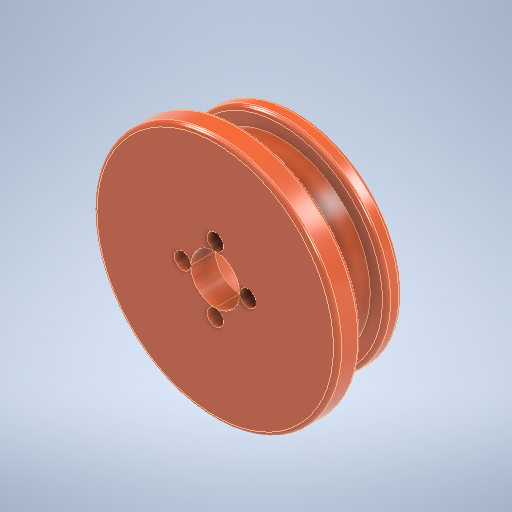
# Autodesk Inventor part: Steering Gear Plate
Saved by Autodesk Inventor 2025.2 (Build 292293000, 293)
## iProperties
Created: 2025-02-06
Part Number: Steering Gear Plate
Material: Generic
Document SubType Name: Modeling
Designer: eason
Density: 1 g/cm^3
Appearance: Smooth - Light Orange
Author: eason
Autodesk Inventor part; units mm, degrees
ref_plane "YZ Plane" through (0, 0, 0) normal (1, 0, 0) x (0, 1, 0)
ref_plane "XZ Plane" through (0, 0, 0) normal (0, 1, 0) x (-1, 0, 0)
sketch "Sketch1" plane through (0, 0, 0) normal (0, 0, 1) x (1, 0, 0)
  circle A0 centre (0, 0) radius 15
  circle A1 centre (0, 0) radius 3
  circle A2 centre (0, 0) radius 5
  circle A3 centre (4, 0) radius 1
  circle A4 centre (-4, 0) radius 1
  line L0 (-21, 0) -> (21, 0) projected
  circle A5 centre (0, 4) radius 1
  circle A6 centre (0, -4) radius 1
  line L1 (0, -21) -> (0, 21) projected
  point P0 (-5, 0)
  point P1 (-3, 0)
  point P2 (3, 0)
  point P3 (5, 0)
  point P4 (0, -5)
  point P5 (0, -3)
  point P6 (0, 3)
  point P7 (0, 5)
  dimension "d0" = 30
  dimension "d1" = 6
  dimension "d2" = 10
  constraints: 8 tangent, 7 centre point, 4 point on line, 3 coincident
  measures "d0" diameter of A0
  measures "d1" diameter of A1
  measures "d2" diameter of A2
extrude "Extrusion1" add sketch "Sketch1" along normal blind 3 contours L0 A2 L1 A0 | A0 L1 A2 L0 | L1 A2 L0 A0 | A0 L0 A2 L1 | A3 A1 A5 A2 | A2 A6 A1 A3 | A5 A1 A4 A2 | A2 A4 A1 A6
ref_plane "Work Plane1" through (0, 0, 1.5) normal (0, 0, 1) x (1, 0, 0)
sketch "Sketch5" plane through (0, 0, 0) normal (0, 0, -1) x (-1, 0, 0)
  line L0 (0, 0) -> (-5.2212, -14.062) construction
  circle A0 centre (0, 0) radius 15 projected
  line L1 (0, -21) -> (0, 21) projected
  circle A1 centre (-4.351, -11.7183) radius 2.5
  arc A2 (-3, 0) -> (3, 0) centre (0, 0) ccw projected
  arc A3 (0.0912, -10.9996) -> (-7.2478, -8.2746) centre (-4.351, -11.7183) ccw
  arc A4 (0.0912, -10.9996) -> (-7.2478, -8.2746) centre (0, 0) ccw
  circle A5 centre (0, 0) radius 8
  point P0 (-2.7846, -7.4997)
  dimension "d25" = 20.37
  dimension "d26" = 5
  dimension "d30" = 2
  dimension "d32" = 4
  constraints: 4 centre point, 4 point on circle, 3 coincident, 2 end point, 1 point on line, 1 tangent, 3 other
  measures "d25" angle of L1 L0
  measures "d26" diameter of A1
  measures "d30" radial gap between concentric circles of A3 A1
extrude "Extrusion5" add sketch "Sketch5" along normal blind 5 contours A1 | A4 A3 L1 A5 | L1 A5 A3 A4 | A3 A5 L1
sketch "Sketch6" plane through (0, 0, -5) normal (0, 0, -1) x (-1, 0, 0)
  arc A0 (-0.0374, -12.9999) -> (-8.4558, -9.8742) centre (0, 0) ccw
  arc A1 (0.0912, -10.9996) -> (-7.2478, -8.2746) centre (0, 0) ccw projected
  arc A2 (-7.2478, -8.2746) -> (-8.4558, -9.8742) centre (-4.351, -11.7183) ccw
  arc A3 (-0.0374, -12.9999) -> (0.0912, -10.9996) centre (-4.351, -11.7183) ccw
  arc A4 (-2.7846, -7.4997) -> (-7.2478, -8.2746) centre (-4.351, -11.7183) ccw projected
  arc A5 (0.0912, -10.9996) -> (-2.7846, -7.4997) centre (-4.351, -11.7183) ccw projected
  arc A6 (-3, 0) -> (3, 0) centre (0, 0) ccw projected
  circle A7 centre (0, 0) radius 8
  circle A8 centre (0, 0) radius 8 projected
  point P0 (-2.7846, -7.4997)
  point P1 (-2.7846, -7.4997)
  dimension "d37" = 2
  constraints: 6 point on circle, 4 centre point, 4 coincident, 2 concentric, 2 other
  measures "d37" radial gap between concentric circles of A0 A1
extrude "Extrusion6" add sketch "Sketch6" along normal blind 2
fillet "Fillet4" radius 0.5 6 edges at (-4.5251, 12.187, -5) (-4.5251, 12.187, -7) (6.851, -11.7183, -5) (12.315, -8.5639, 0) (-12.315, 8.5639, 0) (-15, 0, 3)
body "Solid1"
